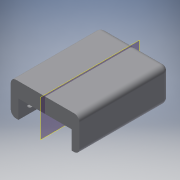
# Autodesk Inventor part: Bottom
Saved by Autodesk Inventor 2018 (Build 220112000, 112)
## iProperties
Created: 2018-05-15
Part Number: Bottom
Material: Generic
Document SubType Name: Modeling
Designer: Mandus
Density: 1 g/cm^3
Appearance: Default
Author: Mandus
Autodesk Inventor part; units mm, degrees
ref_plane "YZ Plane" through (0, 0, 0) normal (1, 0, 0) x (0, 1, 0)
ref_plane "XZ Plane" through (0, 0, 0) normal (0, 1, 0) x (-1, 0, 0)
sketch "Sketch1" plane through (0, 0, 0) normal (0, 0, 1) x (1, 0, 0)
  line L0 (-13, 18.5) -> (13, 18.5)
  line L1 (13, 18.5) -> (13, -15.5)
  line L2 (13, -15.5) -> (-13, -15.5)
  line L3 (-13, -15.5) -> (-13, 18.5)
  line L4 (10, 15.5) -> (-10, 15.5) construction
  line L5 (-10, 15.5) -> (-10, -15.5) construction
  line L6 (10, -15.5) -> (10, 15.5) construction
  line L7 (-10, -15.5) -> (10, -15.5) construction
  point P0 (0, 0)
  point P1 (0, -15.5)
  dimension "d0" = 3
  dimension "d1" = 3
  dimension "d2" = 3
  constraints: 8 end point, 2 parallel, 1 horizontal, 1 horizontal alignment, 1 midpoint, 1 perpendicular
  measures "d0" distance from line of L5 L0.start
  measures "d1" distance from line of L6 L0.end
  measures "d2" distance from line of L4 L0.end
extrude "Extrusion1" add sketch "Sketch1" along normal blind 2
sketch "Sketch2" plane through (0, 0, 0) normal (0, 0, -1) x (-1, 0, 0)
  line L0 (13, -15.5) -> (-13, -15.5) projected
  line L1 (-13, 18.5) -> (13, 18.5) projected
  line L2 (-13, -15.5) -> (13, -15.5)
  line L3 (13, -15.5) -> (13, 18.5)
  line L4 (13, 18.5) -> (-13, 18.5)
  line L5 (-13, 18.5) -> (-13, -15.5)
  line L6 (13, 18.5) -> (-13, 18.5) projected
  line L7 (-8, 18.5) -> (8, 18.5)
  line L8 (8, 18.5) -> (8, -11.5)
  line L9 (8, -11.5) -> (-8, -11.5)
  line L10 (-8, -11.5) -> (-8, 18.5)
  point P0 (0, 0)
  dimension "d5" = 5
  dimension "d6" = 5
  dimension "d7" = 4
  constraints: 16 end point, 4 parallel, 2 horizontal, 2 perpendicular, 1 point on line
  measures "d5" distance from line of L5 L9.end
  measures "d6" distance from line of L3 L8.end
  measures "d7" distance from line of L0 L8.end
extrude "Extrusion2" add sketch "Sketch2" along normal blind 2 contours L0 L5 L1 L10 L9 L8 L3
sketch "Sketch3" plane through (0, 0, 0) normal (0, 0, -1) x (-1, 0, 0)
  line L0 (-13, -15.5) -> (13, -15.5) projected
  line L1 (13, 18.5) -> (13, -15.5) projected
  line L2 (-13, -15.5) -> (13, -15.5)
  line L3 (13, -15.5) -> (13, 18.5)
  line L4 (13, 18.5) -> (-13, 18.5)
  line L5 (-13, 18.5) -> (-13, -15.5)
  line L6 (-10.1, -15.5) -> (10.1, -15.5)
  line L7 (10.1, -15.5) -> (10.1, 15.6)
  line L8 (10.1, 15.6) -> (-10.1, 15.6)
  line L9 (-10.1, 15.6) -> (-10.1, -15.5)
  point P0 (0, 0)
  dimension "d10" = 2.9
  dimension "d11" = 2.9
  dimension "d12" = 2.9
  constraints: 16 end point, 4 parallel, 2 horizontal, 2 perpendicular, 1 point on line
  measures "d10" distance from line of L5 L6.start
  measures "d11" distance from line of L7 L1.start
  measures "d12" distance from line of L8 L4.end
ref_plane "Work Plane1" through (-10, -15.5, -10.7) normal (0, 0, -1) x (0, 1, 0)
extrude "Extrusion3" add sketch "Sketch3" along normal up to surface (10.7 mm away) contours L5 L4 L1 L0 L7 L8 L9
sketch "Sketch4" plane through (10.1, -15.5, -2) normal (-1, 0, 0) x (0, 0, 1)
  arc A0 (-6.7, 5) -> (-3.7, 5) centre (-5.2, 5) ccw construction
  line L0 (-3.7, 5) -> (-3.7, 10) construction
  arc A1 (-3.7, 10) -> (-6.7, 10) centre (-5.2, 10) ccw construction
  line L1 (-6.7, 10) -> (-6.7, 5) construction
  arc A2 (-6.7, 21) -> (-3.7, 21) centre (-5.2, 21) ccw construction
  line L2 (-3.7, 21) -> (-3.7, 26) construction
  arc A3 (-3.7, 26) -> (-6.7, 26) centre (-5.2, 26) ccw construction
  line L3 (-6.7, 26) -> (-6.7, 21) construction
  line L4 (-8.7, 0) -> (-8.7, 31) construction
  line L5 (-8.7, 31) -> (-1.7, 31) construction
  line L6 (-1.7, 0) -> (-1.7, 31) construction
  line L7 (-8.7, 0) -> (-1.7, 0) construction
  arc A4 (-3.4, 10) -> (-7, 10) centre (-5.2, 10) ccw
  line L8 (-3.4, 10) -> (-3.4, 5)
  arc A5 (-7, 5) -> (-3.4, 5) centre (-5.2, 5) ccw
  line L9 (-7, 5) -> (-7, 10)
  arc A6 (-7, 21) -> (-3.4, 21) centre (-5.2, 21) ccw
  line L10 (-7, 21) -> (-7, 26)
  arc A7 (-3.4, 26) -> (-7, 26) centre (-5.2, 26) ccw
  line L11 (-3.4, 26) -> (-3.4, 21)
  point P0 (2, 15.5)
  dimension "d15" = 0.3
  dimension "d16" = 0.3
  constraints: 8 end point, 8 point on circle, 4 centre point, 6 other
  measures "d15" radial gap between concentric circles of A1 A4
  measures "d16" radial gap between concentric circles of A2 A6
extrude "Extrusion4" cut sketch "Sketch4" against normal blind 1.3
ref_plane "Work Plane2" through (0, -15.5, -2) normal (-1, 0, 0) x (0, 0, 1)
mirror "Mirror1" about plane through (0, -15.5, -2) normal (-1, 0, 0) of "Extrusion4"
fillet "Fillet1" radius 2 2 edges at (13, 18.5, -4.35) (-13, 18.5, -4.35)
fillet "Fillet2" radius 2 10 edges at (12.4142, 17.9142, -10.7) (0, 18.5, -10.7) (-12.4142, 17.9142, -10.7) (-13, 0.5, -10.7) (13, 0.5, -10.7) (12.4142, 17.9142, 2) (0, 18.5, 2) (-12.4142, 17.9142, 2) (-13, 0.5, 2) (13, 0.5, 2)
sketch "Sketch5" plane through (0, 0, -2) normal (0, 0, -1) x (-1, 0, 0)
  line L0 (10.1, -15.5) -> (10.1, 15.6) projected
  line L1 (10.1, -15.5) -> (-10.1, -15.5)
  line L2 (-10.1, -15.5) -> (-10.1, -11.5)
  line L3 (-10.1, -11.5) -> (10.1, -11.5)
  line L4 (10.1, -11.5) -> (10.1, -15.5)
  point P0 (0, 0)
  dimension "d21" = 4
  constraints: 8 end point, 2 parallel, 1 horizontal, 1 perpendicular
  measures "d21" distance of L1.end L2.end
extrude "Extrusion5" add sketch "Sketch5" along normal blind 1.7
ref_plane "Work Plane3" through (0, -15.5, -2) normal (-1, 0, 0) x (0, 0, 1)
body "Solid1"
